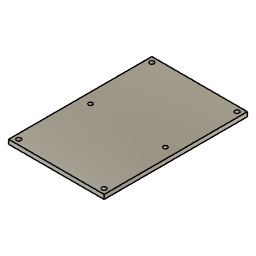
shelf_panel_2 v1 (Autodesk Fusion 360 design; units mm, degrees)
Autodesk Fusion 360 part; units mm, degrees
note: some values were not read from the file. Set by a fixed rule: which sketch regions a step uses.
sketch "Sketch1" plane through (0, 0, 0) normal (0, 0, 1) x (1, 0, 0)
  line L0 (0, 0) -> (140, 0)
  line L1 (140, 0) -> (140, 210)
  line L2 (140, 210) -> (0, 210)
  line L3 (0, 210) -> (0, 0)
  dimension "d1" = 140
  dimension "d2" = 210
  constraint horizontal L0
  constraint vertical L1
  constraint horizontal L2
  constraint vertical L3
  constraint coincident L0.start L3.end
  measures "d1" distance of L0.start L0.end
  measures "d2" distance of L0.start L2.end
extrude "Extrude1" add sketch "Sketch1" along normal blind 6.35
sketch "Sketch2" plane through (0, 0, 6.35) normal (0, 0, 1) x (-1, 0, 0)
  line L0 (0, -210) -> (0, 0)
  line L1 (0, 0) -> (-140, 0)
  line L2 (-140, 0) -> (-140, -210)
  line L3 (-140, -210) -> (0, -210)
  circle A0 centre (-132.5, -7.5) radius 3.2
  line L4 (-140, -105) -> (0, -105)
  line L5 (-70, 0) -> (-70, -210)
  circle A1 centre (-7.5, -7.5) radius 3.2
  circle A2 centre (-132.5, -202.5) radius 3.2
  circle A3 centre (-7.5, -202.5) radius 3.2
  dimension "d5" = 6.4
  dimension "d6" = 7.5
  dimension "d7" = 7.5
  constraint midpoint L2 L4.start
  constraint midpoint L0 L4.end
  constraint midpoint L1 L5.start
  constraint midpoint L3 L5.end
  constraint symmetric A0 L5 A1
  constraint symmetric A0 L4 A2
  constraint symmetric L4 A1 A3
  measures "d5" diameter of A0
  measures "d6" distance of L1 A0.centre
  measures "d7" distance of L2 A0.centre
extrude "Extrude2" cut sketch "Sketch2" against normal blind 10 contours A0 | A1 | A2 | A3
sketch "Sketch3" plane through (0, 0, 6.35) normal (0, 0, 1) x (-1, 0, 0)
  circle A0 centre (-7.5, -7.5) radius 3.2
  circle A1 centre (-7.5, -202.5) radius 3.2
  circle A2 centre (-132.5, -7.5) radius 3.2
  circle A3 centre (-132.5, -202.5) radius 3.2
  line L0 (0, -210) -> (0, 0)
  line L1 (0, 0) -> (-140, 0)
  line L2 (-140, 0) -> (-140, -210)
  line L3 (-140, -210) -> (0, -210)
  line L4 (0, -105) -> (-140, -105)
  circle A4 centre (-15, -105) radius 3
  circle A5 centre (-125, -105) radius 3
  dimension "d10" = 6
  dimension "d11" = 6
  dimension "d12" = 110
  dimension "d13" = 15
  constraint midpoint L0 L4.start
  constraint midpoint L2 L4.end
  constraint coincident L4 A4.centre
  constraint coincident L4 A5.centre
  measures "d10" diameter of A4
  measures "d11" diameter of A5
  measures "d12" distance of A4.centre A5.centre
  measures "d13" distance of L2 A5.centre
extrude "Extrude3" cut sketch "Sketch3" against normal blind 10 contours L4 A4 | L4 A4 | L4 A5 | L4 A5
